Geburtstagsschild (Autodesk Fusion 360 design; units mm, degrees)
Autodesk Fusion 360 part; units mm, degrees
sketch "Sketch2" plane through (0, 0, 0) normal (0, 0, 1) x (1, 0, 0)
  line L0 (0, 0) -> (310, 0)
  line L1 (310, 0) -> (310, 55)
  line L2 (310, 55) -> (0, 55)
  line L3 (0, 55) -> (0, 0)
  dimension "d9" = 310
  dimension "d10" = 55
  constraint horizontal L0
  constraint vertical L1
  constraint horizontal L2
  constraint vertical L3
  constraint coincident L0.start L3.end
  measures "d9" distance of L0.start L0.end
  measures "d10" distance of L0.start L2.end
sketch "Sketch1" plane through (0, 0, 0) normal (0, 0, 1) x (1, 0, 0)
  spline S0 degree 3 poles (59.8411, 26.3898) (55.5097, 27.2397) (53.6137, 32.5028) (55.9347, 36.1804) knots 0 0 0 0 1 1 1 1
  spline S1 degree 3 poles (55.9347, 36.1804) (56.9971, 37.8639) (58.9421, 39.0407) (60.8872, 39.335) knots 0 0 0 0 1 1 1 1
  spline S2 degree 3 poles (60.8872, 39.335) (61.4756, 38.6158) (62.2928, 38.0764) (63.2899, 37.9456) knots 0 0 0 0 1 1 1 1
  spline S3 degree 3 poles (63.2899, 37.9456) (65.2349, 37.7005) (65.856, 39.1225) (64.1071, 39.6782) knots 0 0 0 0 1 1 1 1
  spline S4 degree 3 poles (64.1071, 39.6782) (63.6985, 39.809) (63.1755, 39.907) (62.5707, 39.9561) knots 0 0 0 0 1 1 1 1
  spline S5 degree 3 poles (62.5707, 39.9561) (61.2631, 41.4434) (61.2141, 44.2057) (62.9303, 45.1701) knots 0 0 0 0 1 1 1 1
  spline S6 degree 3 poles (62.9303, 45.1701) (65.856, 46.8373) (66.9021, 43.4212) (65.2022, 43.225) knots 0 0 0 0 1 1 1 1
  spline S7 degree 3 poles (65.2022, 43.225) (64.8753, 43.3721) (64.2542, 43.4048) (64.0254, 43.0943) knots 0 0 0 0 1 1 1 1
  spline S8 degree 3 poles (64.0254, 43.0943) (63.2899, 42.1463) (65.1859, 40.9041) (66.2973, 42.4405) knots 0 0 0 0 1 1 1 1
  spline S9 degree 3 poles (66.2973, 42.4405) (68.2914, 45.1701) (64.7609, 47.442) (61.6881, 45.497) knots 0 0 0 0 1 1 1 1
  spline S10 degree 3 poles (61.6881, 45.497) (59.6286, 44.2057) (59.4815, 41.6723) (60.5112, 39.8907) knots 0 0 0 0 1 1 1 1
  spline S11 degree 3 poles (60.5112, 39.8907) (57.4874, 39.5311) (53.9242, 37.9293) (52.8455, 33.9902) knots 0 0 0 0 1 1 1 1
  spline S12 degree 3 poles (52.8455, 33.9902) (50.3283, 24.7716) (62.8322, 20.7181) (66.232, 29.1357) knots 0 0 0 0 1 1 1 1
  spline S13 degree 3 poles (66.232, 29.1357) (66.706, 30.3126) (66.8367, 32.5355) (65.5291, 33.2547) knots 0 0 0 0 1 1 1 1
  spline S14 degree 3 poles (65.5291, 33.2547) (64.0744, 34.0555) (62.8812, 31.8326) (64.6301, 31.6692) knots 0 0 0 0 1 1 1 1
  spline S15 degree 3 poles (64.6301, 31.6692) (65.4801, 31.3913) (65.856, 30.3616) (65.5291, 29.3809) knots 0 0 0 0 1 1 1 1
  spline S16 degree 3 poles (65.5291, 29.3809) (64.6792, 26.8311) (62.3092, 25.9158) (59.8411, 26.3898) knots 0 0 0 0 1 1 1 1
  spline S17 degree 3 poles (68.7369, 41.9338) (69.3253, 41.7703) (69.9464, 42.2443) (70.1426, 42.9799) knots 0 0 0 0 1 1 1 1
  spline S18 degree 3 poles (70.1426, 42.9799) (70.3224, 43.7154) (69.9955, 44.4509) (69.407, 44.6144) knots 0 0 0 0 1 1 1 1
  spline S19 degree 3 poles (69.407, 44.6144) (68.8186, 44.7778) (68.2139, 44.3201) (68.0014, 43.5846) knots 0 0 0 0 1 1 1 1
  spline S20 degree 3 poles (68.0014, 43.5846) (67.8216, 42.8328) (68.1485, 42.0972) (68.7369, 41.9338) knots 0 0 0 0 1 1 1 1
  spline S21 degree 3 poles (66.0727, 35.0853) (65.6804, 33.794) (66.0727, 32.5028) (67.0861, 32.5028) knots 0 0 0 0 1 1 1 1
  spline S22 degree 3 poles (67.0861, 32.5028) (68.933, 32.5028) (69.8647, 34.8238) (70.3714, 36.7525) knots 0 0 0 0 1 1 1 1
  line L0 (70.3714, 36.7525) -> (69.832, 36.7525)
  spline S23 degree 3 poles (69.832, 36.7525) (69.0311, 34.3171) (68.41, 33.6633) (67.8706, 33.6633) knots 0 0 0 0 1 1 1 1
  spline S24 degree 3 poles (67.8706, 33.6633) (67.4784, 33.6633) (67.5764, 33.9902) (67.7399, 34.5622) knots 0 0 0 0 1 1 1 1
  spline S25 degree 3 poles (67.7399, 34.5622) (67.8543, 34.9382) (69.0965, 39.7599) (69.1782, 40.0378) knots 0 0 0 0 1 1 1 1
  spline S26 degree 3 poles (69.1782, 40.0378) (69.309, 40.5281) (69.1782, 40.806) (68.6715, 40.806) knots 0 0 0 0 1 1 1 1
  line L1 (68.6715, 40.806) -> (67.2495, 40.806)
  spline S27 degree 3 poles (67.2495, 40.806) (67.5764, 40.5118) (67.511, 40.0378) (67.2495, 39.2532) knots 0 0 0 0 1 1 1 1
  spline S28 degree 3 poles (67.2495, 39.2532) (67.1188, 38.8773) (66.1871, 35.4612) (66.0727, 35.0853) knots 0 0 0 0 1 1 1 1
  spline S29 degree 3 poles (73.4638, 32.372) (75.2617, 32.372) (76.2261, 34.8238) (76.8635, 36.7525) knots 0 0 0 0 1 1 1 1
  line L2 (76.8635, 36.7525) -> (76.3732, 36.7525)
  spline S30 degree 3 poles (76.3732, 36.7525) (75.4579, 34.3171) (74.8858, 33.696) (74.4281, 33.696) knots 0 0 0 0 1 1 1 1
  spline S31 degree 3 poles (74.4281, 33.696) (74.0359, 33.696) (73.9868, 33.9902) (74.1176, 34.4315) knots 0 0 0 0 1 1 1 1
  spline S32 degree 3 poles (74.1176, 34.4315) (74.2647, 34.9545) (75.0002, 36.8178) (75.5069, 38.485) knots 0 0 0 0 1 1 1 1
  spline S33 degree 3 poles (75.5069, 38.485) (76.0299, 40.1685) (75.3598, 41.0675) (74.3301, 41.0675) knots 0 0 0 0 1 1 1 1
  spline S34 degree 3 poles (74.3301, 41.0675) (73.5455, 41.0675) (72.7773, 40.5118) (72.1235, 39.4657) knots 0 0 0 0 1 1 1 1
  spline S35 degree 3 poles (72.1235, 39.4657) (72.1725, 40.2993) (71.6332, 40.806) (70.9467, 40.806) knots 0 0 0 0 1 1 1 1
  line L3 (70.9467, 40.806) -> (70.5707, 40.806)
  spline S36 degree 3 poles (70.5707, 40.806) (70.914, 40.4137) (70.7996, 40.0378) (70.5707, 39.2532) knots 0 0 0 0 1 1 1 1
  spline S37 degree 3 poles (70.5707, 39.2532) (70.3909, 38.6158) (69.1487, 34.5296) (68.5767, 32.6335) knots 0 0 0 0 1 1 1 1
  line L4 (68.5767, 32.6335) -> (69.7698, 32.6335)
  spline S38 degree 3 poles (69.7698, 32.6335) (70.2929, 32.6335) (70.5544, 33.0258) (70.6688, 33.5325) knots 0 0 0 0 1 1 1 1
  spline S39 degree 3 poles (70.6688, 33.5325) (70.7505, 33.8758) (71.2245, 35.4449) (71.6332, 36.9649) knots 0 0 0 0 1 1 1 1
  spline S40 degree 3 poles (71.6332, 36.9649) (72.287, 38.91) (73.1205, 40.1685) (73.807, 40.1685) knots 0 0 0 0 1 1 1 1
  spline S41 degree 3 poles (73.807, 40.1685) (74.183, 40.1685) (74.3301, 39.7763) (74.0849, 39.0081) knots 0 0 0 0 1 1 1 1
  spline S42 degree 3 poles (74.0849, 39.0081) (73.807, 38.1091) (72.9081, 36.3765) (72.4177, 34.8238) knots 0 0 0 0 1 1 1 1
  spline S43 degree 3 poles (72.4177, 34.8238) (72.0091, 33.5489) (72.4504, 32.372) (73.4638, 32.372) knots 0 0 0 0 1 1 1 1
  line L5 (77.6468, 26.7494) -> (79.1178, 26.7494)
  spline S44 degree 3 poles (79.1178, 26.7494) (79.6409, 26.7494) (79.9024, 27.1417) (80.0168, 27.6483) knots 0 0 0 0 1 1 1 1
  spline S45 degree 3 poles (80.0168, 27.6483) (80.0822, 27.9099) (80.7523, 30.3616) (81.4715, 32.9604) knots 0 0 0 0 1 1 1 1
  spline S46 degree 3 poles (81.4715, 32.9604) (81.7004, 32.6662) (82.0599, 32.5028) (82.583, 32.5028) knots 0 0 0 0 1 1 1 1
  spline S47 degree 3 poles (82.583, 32.5028) (84.152, 32.5028) (85.7538, 34.4805) (86.3749, 36.7525) knots 0 0 0 0 1 1 1 1
  spline S48 degree 3 poles (86.3749, 36.7525) (87.045, 39.2369) (86.7672, 41.0675) (85.1817, 41.0675) knots 0 0 0 0 1 1 1 1
  spline S49 degree 3 poles (85.1817, 41.0675) (84.3481, 41.0675) (83.6291, 40.4301) (83.0243, 39.4003) knots 0 0 0 0 1 1 1 1
  spline S50 degree 3 poles (83.0243, 39.4003) (83.1224, 40.283) (82.5666, 40.806) (81.8638, 40.806) knots 0 0 0 0 1 1 1 1
  line L6 (81.8638, 40.806) -> (81.4879, 40.806)
  spline S51 degree 3 poles (81.4879, 40.806) (81.8148, 40.4628) (81.7167, 40.0378) (81.4879, 39.2532) knots 0 0 0 0 1 1 1 1
  spline S52 degree 3 poles (81.4879, 39.2532) (81.259, 38.4687) (78.415, 28.4329) (78.2189, 27.7791) knots 0 0 0 0 1 1 1 1
  spline S53 degree 3 poles (78.2189, 27.7791) (78.0391, 27.158) (77.9083, 26.8801) (77.6468, 26.7494) knots 0 0 0 0 1 1 1 1
  line L7 (81.6677, 33.6633) -> (82.4032, 36.3765)
  spline S54 degree 3 poles (82.4032, 36.3765) (82.9753, 38.3706) (83.7435, 39.8907) (84.3972, 40.0378) knots 0 0 0 0 1 1 1 1
  spline S55 degree 3 poles (84.3972, 40.0378) (85.0673, 40.1849) (85.1, 39.1552) (84.5606, 37.1447) knots 0 0 0 0 1 1 1 1
  spline S56 degree 3 poles (84.5606, 37.1447) (84.0703, 35.3468) (83.4329, 33.794) (82.4686, 33.3527) knots 0 0 0 0 1 1 1 1
  spline S57 degree 3 poles (82.4686, 33.3527) (82.0926, 33.1729) (81.7984, 33.32) (81.6677, 33.6633) knots 0 0 0 0 1 1 1 1
  spline S58 degree 3 poles (88.2614, 32.372) (89.0296, 32.372) (89.7161, 33.0422) (90.2554, 33.9738) knots 0 0 0 0 1 1 1 1
  spline S59 degree 3 poles (90.2554, 33.9738) (90.2881, 33.1402) (90.6968, 32.5028) (91.4159, 32.5028) knots 0 0 0 0 1 1 1 1
  spline S60 degree 3 poles (91.4159, 32.5028) (93.0995, 32.5028) (94.0311, 34.8238) (94.5378, 36.7525) knots 0 0 0 0 1 1 1 1
  line L8 (94.5378, 36.7525) -> (93.9984, 36.7525)
  spline S61 degree 3 poles (93.9984, 36.7525) (93.1975, 34.3171) (92.5764, 33.6633) (92.2005, 33.6633) knots 0 0 0 0 1 1 1 1
  spline S62 degree 3 poles (92.2005, 33.6633) (91.8082, 33.6633) (91.8082, 33.9902) (91.9717, 34.5622) knots 0 0 0 0 1 1 1 1
  spline S63 degree 3 poles (91.9717, 34.5622) (92.0697, 34.9055) (93.3283, 39.7109) (93.6061, 40.806) knots 0 0 0 0 1 1 1 1
  line L9 (93.6061, 40.806) -> (92.0534, 40.806)
  spline S64 degree 3 poles (92.0534, 40.806) (92.0043, 40.7079) (91.9226, 40.4301) (91.8082, 40.0378) knots 0 0 0 0 1 1 1 1
  spline S65 degree 3 poles (91.8082, 40.0378) (91.7101, 40.6099) (91.4159, 41.0512) (90.8275, 41.0512) knots 0 0 0 0 1 1 1 1
  spline S66 degree 3 poles (90.8275, 41.0512) (89.8959, 41.0512) (88.1633, 39.6292) (87.3134, 36.7851) knots 0 0 0 0 1 1 1 1
  spline S67 degree 3 poles (87.3134, 36.7851) (86.4634, 33.9411) (87.1336, 32.372) (88.2614, 32.372) knots 0 0 0 0 1 1 1 1
  spline S68 degree 3 poles (88.9479, 36.7525) (89.5036, 38.7302) (90.5333, 39.9397) (91.0563, 39.9397) knots 0 0 0 0 1 1 1 1
  spline S69 degree 3 poles (91.0563, 39.9397) (91.5303, 39.9397) (91.563, 39.335) (91.465, 38.8773) knots 0 0 0 0 1 1 1 1
  spline S70 degree 3 poles (91.465, 38.8773) (91.0727, 37.488) (90.5987, 35.7881) (90.4516, 35.2487) knots 0 0 0 0 1 1 1 1
  spline S71 degree 3 poles (90.4516, 35.2487) (90.2064, 34.6113) (89.8305, 33.9738) (89.3401, 33.9738) knots 0 0 0 0 1 1 1 1
  spline S72 degree 3 poles (89.3401, 33.9738) (88.7517, 33.9738) (88.4412, 34.9382) (88.9479, 36.7525) knots 0 0 0 0 1 1 1 1
  spline S73 degree 3 poles (94.9495, 32.372) (95.7177, 32.372) (96.4042, 33.0422) (96.9436, 33.9738) knots 0 0 0 0 1 1 1 1
  spline S74 degree 3 poles (96.9436, 33.9738) (96.9763, 33.1402) (97.3849, 32.5028) (98.1041, 32.5028) knots 0 0 0 0 1 1 1 1
  spline S75 degree 3 poles (98.1041, 32.5028) (99.7876, 32.5028) (100.7192, 34.8238) (101.2259, 36.7525) knots 0 0 0 0 1 1 1 1
  line L10 (101.2259, 36.7525) -> (100.6866, 36.7525)
  spline S76 degree 3 poles (100.6866, 36.7525) (99.8857, 34.3171) (99.2646, 33.6633) (98.8886, 33.6633) knots 0 0 0 0 1 1 1 1
  spline S77 degree 3 poles (98.8886, 33.6633) (98.4963, 33.6633) (98.4963, 33.9902) (98.6598, 34.5622) knots 0 0 0 0 1 1 1 1
  spline S78 degree 3 poles (98.6598, 34.5622) (98.7579, 34.9055) (100.0164, 39.7109) (100.2943, 40.806) knots 0 0 0 0 1 1 1 1
  line L11 (100.2943, 40.806) -> (98.7415, 40.806)
  spline S79 degree 3 poles (98.7415, 40.806) (98.6925, 40.7079) (98.6108, 40.4301) (98.4963, 40.0378) knots 0 0 0 0 1 1 1 1
  spline S80 degree 3 poles (98.4963, 40.0378) (98.3983, 40.6099) (98.1041, 41.0512) (97.5156, 41.0512) knots 0 0 0 0 1 1 1 1
  spline S81 degree 3 poles (97.5156, 41.0512) (96.584, 41.0512) (94.8514, 39.6292) (94.0015, 36.7851) knots 0 0 0 0 1 1 1 1
  spline S82 degree 3 poles (94.0015, 36.7851) (93.1516, 33.9411) (93.8217, 32.372) (94.9495, 32.372) knots 0 0 0 0 1 1 1 1
  spline S83 degree 3 poles (95.636, 36.7525) (96.1917, 38.7302) (97.2214, 39.9397) (97.7445, 39.9397) knots 0 0 0 0 1 1 1 1
  spline S84 degree 3 poles (97.7445, 39.9397) (98.2185, 39.9397) (98.2512, 39.335) (98.1531, 38.8773) knots 0 0 0 0 1 1 1 1
  spline S85 degree 3 poles (98.1531, 38.8773) (97.7608, 37.488) (97.2868, 35.7881) (97.1397, 35.2487) knots 0 0 0 0 1 1 1 1
  spline S86 degree 3 poles (97.1397, 35.2487) (96.8945, 34.6113) (96.5186, 33.9738) (96.0283, 33.9738) knots 0 0 0 0 1 1 1 1
  spline S87 degree 3 poles (96.0283, 33.9738) (95.4398, 33.9738) (95.1293, 34.9382) (95.636, 36.7525) knots 0 0 0 0 1 1 1 1
  line L12 (99.1692, 32.6335) -> (100.6402, 32.6335)
  spline S88 degree 3 poles (100.6402, 32.6335) (101.1633, 32.6335) (101.4248, 33.0258) (101.5392, 33.5325) knots 0 0 0 0 1 1 1 1
  spline S89 degree 3 poles (101.5392, 33.5325) (101.6209, 33.8758) (102.0949, 35.4612) (102.5199, 36.9976) knots 0 0 0 0 1 1 1 1
  spline S90 degree 3 poles (102.5199, 36.9976) (103.1247, 38.8446) (103.4352, 39.3023) (103.8275, 39.6945) knots 0 0 0 0 1 1 1 1
  spline S91 degree 3 poles (103.8275, 39.6945) (104.089, 39.9561) (104.2361, 39.8743) (104.2525, 39.6455) knots 0 0 0 0 1 1 1 1
  spline S92 degree 3 poles (104.2525, 39.6455) (104.3015, 38.959) (105.3149, 38.8119) (105.6745, 39.5474) knots 0 0 0 0 1 1 1 1
  spline S93 degree 3 poles (105.6745, 39.5474) (106.0504, 40.3156) (105.5601, 41.1165) (104.7918, 41.0839) knots 0 0 0 0 1 1 1 1
  spline S94 degree 3 poles (104.7918, 41.0839) (104.1381, 41.0512) (103.5823, 40.5445) (102.9939, 39.4657) knots 0 0 0 0 1 1 1 1
  spline S95 degree 3 poles (102.9939, 39.4657) (103.0429, 40.2993) (102.5036, 40.806) (101.8171, 40.806) knots 0 0 0 0 1 1 1 1
  line L13 (101.8171, 40.806) -> (101.4411, 40.806)
  spline S96 degree 3 poles (101.4411, 40.806) (101.7354, 40.4791) (101.67, 40.0378) (101.4411, 39.2532) knots 0 0 0 0 1 1 1 1
  spline S97 degree 3 poles (101.4411, 39.2532) (101.2123, 38.4687) (99.9374, 34.3171) (99.7413, 33.6633) knots 0 0 0 0 1 1 1 1
  spline S98 degree 3 poles (99.7413, 33.6633) (99.5615, 33.0422) (99.4307, 32.7643) (99.1692, 32.6335) knots 0 0 0 0 1 1 1 1
  spline S99 degree 3 poles (110.832, 24.9024) (117.8603, 24.1015) (124.0223, 35.0362) (124.8722, 42.3914) knots 0 0 0 0 1 1 1 1
  spline S100 degree 3 poles (124.8722, 42.3914) (125.4607, 39.809) (126.0981, 37.2592) (126.3106, 34.6767) knots 0 0 0 0 1 1 1 1
  spline S101 degree 3 poles (126.3106, 34.6767) (125.6078, 33.32) (125.1011, 31.9307) (124.9703, 30.6885) knots 0 0 0 0 1 1 1 1
  spline S102 degree 3 poles (124.9703, 30.6885) (124.6598, 27.7955) (126.5558, 27.8281) (127.2586, 29.953) knots 0 0 0 0 1 1 1 1
  spline S103 degree 3 poles (127.2586, 29.953) (127.798, 31.6038) (127.9941, 34.0555) (127.9941, 36.2131) knots 0 0 0 0 1 1 1 1
  spline S104 degree 3 poles (127.9941, 36.2131) (129.5959, 38.5994) (131.9986, 41.2473) (134.483, 43.4212) knots 0 0 0 0 1 1 1 1
  spline S105 degree 3 poles (134.483, 43.4212) (133.9764, 42.6203) (133.061, 41.5742) (132.015, 39.2859) knots 0 0 0 0 1 1 1 1
  spline S106 degree 3 poles (132.015, 39.2859) (131.1977, 37.488) (131.0016, 35.7227) (131.2141, 33.7123) knots 0 0 0 0 1 1 1 1
  spline S107 degree 3 poles (131.2141, 33.7123) (131.59, 30.051) (134.8426, 27.5176) (137.229, 29.4463) knots 0 0 0 0 1 1 1 1
  spline S108 degree 3 poles (137.229, 29.4463) (138.226, 30.2635) (136.8857, 31.5548) (136.2646, 30.6068) knots 0 0 0 0 1 1 1 1
  spline S109 degree 3 poles (136.2646, 30.6068) (135.8397, 29.9693) (135.2513, 29.577) (134.6465, 29.7242) knots 0 0 0 0 1 1 1 1
  spline S110 degree 3 poles (134.6465, 29.7242) (133.4043, 30.0347) (132.8159, 31.6202) (133.061, 34.6276) knots 0 0 0 0 1 1 1 1
  spline S111 degree 3 poles (133.061, 34.6276) (133.4697, 39.6292) (136.1339, 45.8239) (140.9883, 47.8016) knots 0 0 0 0 1 1 1 1
  spline S112 degree 3 poles (140.9883, 47.8016) (143.6689, 48.8967) (146.0716, 47.6218) (145.1889, 45.971) knots 0 0 0 0 1 1 1 1
  spline S113 degree 3 poles (145.1889, 45.971) (144.9928, 45.6114) (144.0938, 46.1181) (143.2112, 45.4643) knots 0 0 0 0 1 1 1 1
  spline S114 degree 3 poles (143.2112, 45.4643) (142.1325, 44.6634) (143.2439, 42.8328) (145.4178, 44.2057) knots 0 0 0 0 1 1 1 1
  spline S115 degree 3 poles (145.4178, 44.2057) (146.611, 44.9576) (147.1176, 47.1151) (145.8754, 48.1449) knots 0 0 0 0 1 1 1 1
  spline S116 degree 3 poles (145.8754, 48.1449) (144.6002, 49.1746) (142.8353, 49.0602) (141.3806, 48.5698) knots 0 0 0 0 1 1 1 1
  spline S117 degree 3 poles (141.3806, 48.5698) (136.33, 47.2622) (130.6256, 41.1492) (127.9778, 37.4226) knots 0 0 0 0 1 1 1 1
  line L14 (127.9778, 37.4226) -> (127.9778, 37.4716)
  spline S118 degree 3 poles (127.9778, 37.4716) (127.9124, 39.433) (127.4711, 41.4598) (126.6698, 43.2087) knots 0 0 0 0 1 1 1 1
  spline S119 degree 3 poles (126.6698, 43.2087) (123.6464, 49.8284) (116.945, 49.289) (114.5423, 47.0988) knots 0 0 0 0 1 1 1 1
  spline S120 degree 3 poles (114.5423, 47.0988) (111.1916, 44.0586) (113.3327, 37.8312) (118.5795, 39.3513) knots 0 0 0 0 1 1 1 1
  spline S121 degree 3 poles (118.5795, 39.3513) (121.4071, 40.1685) (119.3477, 43.2414) (117.7786, 41.3454) knots 0 0 0 0 1 1 1 1
  spline S122 degree 3 poles (117.7786, 41.3454) (117.2882, 40.7406) (116.7815, 40.5445) (116.1604, 40.6099) knots 0 0 0 0 1 1 1 1
  spline S123 degree 3 poles (116.1604, 40.6099) (113.3327, 40.8877) (113.0385, 45.0393) (115.1634, 46.6248) knots 0 0 0 0 1 1 1 1
  spline S124 degree 3 poles (115.1634, 46.6248) (118.3506, 49.0111) (122.7964, 47.4584) (124.4309, 43.7317) knots 0 0 0 0 1 1 1 1
  spline S125 degree 3 poles (124.4309, 43.7317) (124.4473, 43.225) (124.3982, 42.702) (124.3165, 42.2117) knots 0 0 0 0 1 1 1 1
  spline S126 degree 3 poles (124.3165, 42.2117) (123.3849, 36.3275) (118.2362, 25.3764) (110.9954, 26.8475) knots 0 0 0 0 1 1 1 1
  spline S127 degree 3 poles (110.9954, 26.8475) (109.7202, 27.109) (109.5567, 25.0495) (110.832, 24.9024) knots 0 0 0 0 1 1 1 1
  spline S128 degree 3 poles (125.7058, 29.2828) (125.428, 30.3943) (125.7058, 31.8) (126.3756, 33.3364) knots 0 0 0 0 1 1 1 1
  line L15 (126.3756, 33.3364) -> (126.3756, 33.1893)
  spline S129 degree 3 poles (126.3756, 33.1893) (126.3923, 31.9307) (126.3433, 30.3453) (125.7058, 29.2828) knots 0 0 0 0 1 1 1 1
  spline S130 degree 3 poles (136.913, 32.372) (137.6812, 32.372) (138.3677, 33.0422) (138.9071, 33.9738) knots 0 0 0 0 1 1 1 1
  spline S131 degree 3 poles (138.9071, 33.9738) (138.9398, 33.1402) (139.3484, 32.5028) (140.0676, 32.5028) knots 0 0 0 0 1 1 1 1
  spline S132 degree 3 poles (140.0676, 32.5028) (141.7511, 32.5028) (142.6827, 34.8238) (143.1894, 36.7525) knots 0 0 0 0 1 1 1 1
  line L16 (143.1894, 36.7525) -> (142.65, 36.7525)
  spline S133 degree 3 poles (142.65, 36.7525) (141.8491, 34.3171) (141.228, 33.6633) (140.8521, 33.6633) knots 0 0 0 0 1 1 1 1
  spline S134 degree 3 poles (140.8521, 33.6633) (140.4598, 33.6633) (140.4598, 33.9902) (140.6233, 34.5622) knots 0 0 0 0 1 1 1 1
  spline S135 degree 3 poles (140.6233, 34.5622) (140.7213, 34.9055) (141.9799, 39.7109) (142.2578, 40.806) knots 0 0 0 0 1 1 1 1
  line L17 (142.2578, 40.806) -> (140.705, 40.806)
  spline S136 degree 3 poles (140.705, 40.806) (140.656, 40.7079) (140.5742, 40.4301) (140.4598, 40.0378) knots 0 0 0 0 1 1 1 1
  spline S137 degree 3 poles (140.4598, 40.0378) (140.3618, 40.6099) (140.0676, 41.0512) (139.4791, 41.0512) knots 0 0 0 0 1 1 1 1
  spline S138 degree 3 poles (139.4791, 41.0512) (138.5475, 41.0512) (136.8149, 39.6292) (135.965, 36.7851) knots 0 0 0 0 1 1 1 1
  spline S139 degree 3 poles (135.965, 36.7851) (135.115, 33.9411) (135.7852, 32.372) (136.913, 32.372) knots 0 0 0 0 1 1 1 1
  spline S140 degree 3 poles (137.5995, 36.7525) (138.1552, 38.7302) (139.1849, 39.9397) (139.708, 39.9397) knots 0 0 0 0 1 1 1 1
  spline S141 degree 3 poles (139.708, 39.9397) (140.182, 39.9397) (140.2147, 39.335) (140.1166, 38.8773) knots 0 0 0 0 1 1 1 1
  spline S142 degree 3 poles (140.1166, 38.8773) (139.7243, 37.488) (139.2503, 35.7881) (139.1032, 35.2487) knots 0 0 0 0 1 1 1 1
  spline S143 degree 3 poles (139.1032, 35.2487) (138.858, 34.6113) (138.4821, 33.9738) (137.9917, 33.9738) knots 0 0 0 0 1 1 1 1
  spline S144 degree 3 poles (137.9917, 33.9738) (137.4033, 33.9738) (137.0928, 34.9382) (137.5995, 36.7525) knots 0 0 0 0 1 1 1 1
  spline S145 degree 3 poles (137.8773, 43.127) (137.8773, 42.5222) (138.384, 41.9828) (138.9888, 41.9828) knots 0 0 0 0 1 1 1 1
  spline S146 degree 3 poles (138.9888, 41.9828) (139.5936, 41.9828) (140.1656, 42.5386) (140.1656, 43.176) knots 0 0 0 0 1 1 1 1
  spline S147 degree 3 poles (140.1656, 43.176) (140.1656, 43.8135) (139.5936, 44.2548) (138.9888, 44.2548) knots 0 0 0 0 1 1 1 1
  spline S148 degree 3 poles (138.9888, 44.2548) (138.384, 44.2548) (137.8773, 43.7481) (137.8773, 43.127) knots 0 0 0 0 1 1 1 1
  spline S149 degree 3 poles (140.754, 43.127) (140.754, 42.5222) (141.2607, 41.9992) (141.8655, 41.9992) knots 0 0 0 0 1 1 1 1
  spline S150 degree 3 poles (141.8655, 41.9992) (142.5356, 41.9992) (142.9933, 42.5549) (142.9933, 43.1433) knots 0 0 0 0 1 1 1 1
  spline S151 degree 3 poles (142.9933, 43.1433) (142.9933, 43.8135) (142.4539, 44.2548) (141.8655, 44.2548) knots 0 0 0 0 1 1 1 1
  spline S152 degree 3 poles (141.8655, 44.2548) (141.2444, 44.2548) (140.754, 43.7481) (140.754, 43.127) knots 0 0 0 0 1 1 1 1
  spline S153 degree 3 poles (143.6011, 32.5028) (144.4184, 32.5028) (145.0722, 33.0422) (145.6115, 33.9411) knots 0 0 0 0 1 1 1 1
  spline S154 degree 3 poles (145.6115, 33.9411) (145.6606, 33.1239) (146.0692, 32.5028) (146.772, 32.5028) knots 0 0 0 0 1 1 1 1
  spline S155 degree 3 poles (146.772, 32.5028) (148.4555, 32.5028) (149.3872, 34.8238) (149.8939, 36.7525) knots 0 0 0 0 1 1 1 1
  line L18 (149.8939, 36.7525) -> (149.3545, 36.7525)
  spline S156 degree 3 poles (149.3545, 36.7525) (148.5536, 34.3171) (147.9325, 33.6633) (147.5566, 33.6633) knots 0 0 0 0 1 1 1 1
  spline S157 degree 3 poles (147.5566, 33.6633) (147.1643, 33.6633) (147.2624, 33.9902) (147.4258, 34.5622) knots 0 0 0 0 1 1 1 1
  spline S158 degree 3 poles (147.4258, 34.5622) (147.5402, 34.9382) (148.7824, 39.7599) (148.8642, 40.0378) knots 0 0 0 0 1 1 1 1
  spline S159 degree 3 poles (148.8642, 40.0378) (148.9949, 40.5281) (148.8642, 40.806) (148.3575, 40.806) knots 0 0 0 0 1 1 1 1
  line L19 (148.3575, 40.806) -> (146.9355, 40.806)
  spline S160 degree 3 poles (146.9355, 40.806) (147.2624, 40.4464) (147.197, 40.0378) (146.9355, 39.2532) knots 0 0 0 0 1 1 1 1
  spline S161 degree 3 poles (146.9355, 39.2532) (146.8701, 39.0571) (146.5922, 38.0437) (146.3144, 37.063) knots 0 0 0 0 1 1 1 1
  spline S162 degree 3 poles (146.3144, 37.063) (145.4317, 34.219) (144.925, 33.6633) (144.3203, 33.6633) knots 0 0 0 0 1 1 1 1
  spline S163 degree 3 poles (144.3203, 33.6633) (143.928, 33.6633) (143.6665, 33.9902) (143.8299, 34.5622) knots 0 0 0 0 1 1 1 1
  spline S164 degree 3 poles (143.8299, 34.5622) (143.9444, 34.9382) (145.1866, 39.7599) (145.2683, 40.0378) knots 0 0 0 0 1 1 1 1
  spline S165 degree 3 poles (145.2683, 40.0378) (145.399, 40.5281) (145.2683, 40.806) (144.7616, 40.806) knots 0 0 0 0 1 1 1 1
  line L20 (144.7616, 40.806) -> (143.3396, 40.806)
  spline S166 degree 3 poles (143.3396, 40.806) (143.6665, 40.4464) (143.6011, 40.0378) (143.3396, 39.2532) knots 0 0 0 0 1 1 1 1
  spline S167 degree 3 poles (143.3396, 39.2532) (143.2088, 38.8773) (142.2772, 35.4612) (142.1628, 35.0853) knots 0 0 0 0 1 1 1 1
  spline S168 degree 3 poles (142.1628, 35.0853) (141.7705, 33.794) (142.1628, 32.5028) (143.6011, 32.5028) knots 0 0 0 0 1 1 1 1
  spline S169 degree 3 poles (150.9424, 32.3884) (152.6422, 32.3884) (153.8027, 33.8594) (153.7046, 35.2487) knots 0 0 0 0 1 1 1 1
  spline S170 degree 3 poles (153.7046, 35.2487) (153.5739, 37.063) (152.0702, 38.0764) (151.825, 39.1878) knots 0 0 0 0 1 1 1 1
  spline S171 degree 3 poles (151.825, 39.1878) (151.6125, 40.1522) (152.1028, 40.757) (152.6749, 40.7079) knots 0 0 0 0 1 1 1 1
  spline S172 degree 3 poles (152.6749, 40.7079) (153.2143, 40.6589) (153.2306, 39.9887) (153.1162, 39.4003) knots 0 0 0 0 1 1 1 1
  spline S173 degree 3 poles (153.1162, 39.4003) (152.8874, 38.1908) (154.8324, 38.2235) (154.5873, 39.6945) knots 0 0 0 0 1 1 1 1
  spline S174 degree 3 poles (154.5873, 39.6945) (154.4238, 40.6589) (153.6556, 41.1656) (152.5442, 41.1819) knots 0 0 0 0 1 1 1 1
  spline S175 degree 3 poles (152.5442, 41.1819) (151.4327, 41.1983) (150.1088, 40.283) (150.3703, 38.5014) knots 0 0 0 0 1 1 1 1
  spline S176 degree 3 poles (150.3703, 38.5014) (150.5991, 36.9323) (152.3971, 35.7718) (152.1846, 34.2353) knots 0 0 0 0 1 1 1 1
  spline S177 degree 3 poles (152.1846, 34.2353) (152.0538, 33.3527) (151.5798, 33.0095) (150.9587, 33.0095) knots 0 0 0 0 1 1 1 1
  spline S178 degree 3 poles (150.9587, 33.0095) (149.8473, 33.0095) (149.3242, 34.1209) (150.1741, 35.5429) knots 0 0 0 0 1 1 1 1
  spline S179 degree 3 poles (150.1741, 35.5429) (150.926, 36.7851) (149.2098, 37.3736) (148.7521, 36.1314) knots 0 0 0 0 1 1 1 1
  spline S180 degree 3 poles (148.7521, 36.1314) (148.2291, 34.7093) (148.7031, 32.3884) (150.9424, 32.3884) knots 0 0 0 0 1 1 1 1
  spline S181 degree 3 poles (156.7942, 32.5028) (158.5758, 32.5028) (160.1939, 34.3824) (160.815, 36.7525) knots 0 0 0 0 1 1 1 1
  line L21 (160.815, 36.7525) -> (160.2756, 36.7525)
  spline S182 degree 3 poles (160.2756, 36.7525) (159.4911, 34.3498) (158.2325, 33.5325) (157.3499, 33.696) knots 0 0 0 0 1 1 1 1
  spline S183 degree 3 poles (157.3499, 33.696) (156.549, 33.8431) (156.1567, 35.0362) (156.3855, 36.3765) knots 0 0 0 0 1 1 1 1
  spline S184 degree 3 poles (156.3855, 36.3765) (160.1612, 36.0169) (161.24, 41.0675) (158.5758, 41.0675) knots 0 0 0 0 1 1 1 1
  spline S185 degree 3 poles (158.5758, 41.0675) (156.6798, 41.0675) (155.1597, 38.6812) (154.7674, 36.7198) knots 0 0 0 0 1 1 1 1
  spline S186 degree 3 poles (154.7674, 36.7198) (154.2934, 34.3824) (154.9635, 32.5028) (156.7942, 32.5028) knots 0 0 0 0 1 1 1 1
  spline S187 degree 3 poles (156.4836, 36.8669) (156.974, 38.91) (158.02, 40.5445) (158.8373, 40.5445) knots 0 0 0 0 1 1 1 1
  spline S188 degree 3 poles (158.8373, 40.5445) (159.6055, 40.5445) (158.919, 37.2428) (156.4836, 36.8669) knots 0 0 0 0 1 1 1 1
  spline S189 degree 3 poles (76.4934, 3.3435) (77.7847, 3.3435) (79.2067, 4.6511) (79.7624, 6.7596) knots 0 0 0 0 1 1 1 1
  spline S190 degree 3 poles (79.7624, 6.7596) (80.1547, 7.9201) (81.2661, 12.9053) (81.8872, 15.6348) knots 0 0 0 0 1 1 1 1
  line L22 (81.8872, 15.6348) -> (82.9987, 15.6348)
  line L23 (82.9987, 15.6348) -> (83.1621, 16.2886)
  line L24 (83.1621, 16.2886) -> (82.0507, 16.2886)
  line L25 (82.0507, 16.2886) -> (82.2795, 17.2693)
  spline S191 degree 3 poles (82.2795, 17.2693) (82.6554, 18.7404) (83.2112, 19.5576) (83.8813, 19.8355) knots 0 0 0 0 1 1 1 1
  spline S192 degree 3 poles (83.8813, 19.8355) (84.2409, 19.9826) (84.4207, 19.7701) (84.1591, 19.4269) knots 0 0 0 0 1 1 1 1
  spline S193 degree 3 poles (84.1591, 19.4269) (83.6525, 18.7731) (84.7149, 18.0049) (85.1562, 18.8548) knots 0 0 0 0 1 1 1 1
  spline S194 degree 3 poles (85.1562, 18.8548) (85.4994, 19.5249) (85.0091, 20.4076) (83.8323, 20.4076) knots 0 0 0 0 1 1 1 1
  spline S195 degree 3 poles (83.8323, 20.4076) (82.541, 20.4076) (81.2334, 19.3288) (80.6777, 17.2203) knots 0 0 0 0 1 1 1 1
  spline S196 degree 3 poles (80.6777, 17.2203) (80.6287, 17.0405) (80.5633, 16.7463) (80.4489, 16.2886) knots 0 0 0 0 1 1 1 1
  line L26 (80.4489, 16.2886) -> (79.648, 16.2886)
  line L27 (79.648, 16.2886) -> (79.4845, 15.6348)
  line L28 (79.4845, 15.6348) -> (80.2854, 15.6348)
  spline S197 degree 3 poles (80.2854, 15.6348) (79.9095, 14.1148) (79.2394, 11.3852) (77.9808, 6.4817) knots 0 0 0 0 1 1 1 1
  spline S198 degree 3 poles (77.9808, 6.4817) (77.6049, 5.0107) (77.1145, 4.1934) (76.4444, 3.9156) knots 0 0 0 0 1 1 1 1
  spline S199 degree 3 poles (76.4444, 3.9156) (76.0848, 3.7684) (75.905, 3.9809) (76.1665, 4.3242) knots 0 0 0 0 1 1 1 1
  spline S200 degree 3 poles (76.1665, 4.3242) (76.6732, 4.978) (75.6108, 5.7462) (75.1695, 4.8963) knots 0 0 0 0 1 1 1 1
  spline S201 degree 3 poles (75.1695, 4.8963) (74.8262, 4.2261) (75.3166, 3.3435) (76.4934, 3.3435) knots 0 0 0 0 1 1 1 1
  spline S202 degree 3 poles (83.401, 7.9854) (84.2184, 7.9854) (84.8722, 8.5248) (85.4116, 9.4238) knots 0 0 0 0 1 1 1 1
  spline S203 degree 3 poles (85.4116, 9.4238) (85.4606, 8.6065) (85.8692, 7.9854) (86.5721, 7.9854) knots 0 0 0 0 1 1 1 1
  spline S204 degree 3 poles (86.5721, 7.9854) (88.2556, 7.9854) (89.1872, 10.3064) (89.6939, 12.2351) knots 0 0 0 0 1 1 1 1
  line L29 (89.6939, 12.2351) -> (89.1545, 12.2351)
  spline S205 degree 3 poles (89.1545, 12.2351) (88.3536, 9.7997) (87.7325, 9.1459) (87.3566, 9.1459) knots 0 0 0 0 1 1 1 1
  spline S206 degree 3 poles (87.3566, 9.1459) (86.9643, 9.1459) (87.0624, 9.4728) (87.2258, 10.0449) knots 0 0 0 0 1 1 1 1
  spline S207 degree 3 poles (87.2258, 10.0449) (87.3403, 10.4208) (88.5825, 15.2426) (88.6642, 15.5204) knots 0 0 0 0 1 1 1 1
  spline S208 degree 3 poles (88.6642, 15.5204) (88.795, 16.0108) (88.6642, 16.2886) (88.1575, 16.2886) knots 0 0 0 0 1 1 1 1
  line L30 (88.1575, 16.2886) -> (86.7355, 16.2886)
  spline S209 degree 3 poles (86.7355, 16.2886) (87.0624, 15.9291) (86.997, 15.5204) (86.7355, 14.7359) knots 0 0 0 0 1 1 1 1
  spline S210 degree 3 poles (86.7355, 14.7359) (86.6701, 14.5397) (86.3923, 13.5264) (86.1144, 12.5457) knots 0 0 0 0 1 1 1 1
  spline S211 degree 3 poles (86.1144, 12.5457) (85.2318, 9.7016) (84.7251, 9.1459) (84.1203, 9.1459) knots 0 0 0 0 1 1 1 1
  spline S212 degree 3 poles (84.1203, 9.1459) (83.7279, 9.1459) (83.4664, 9.4728) (83.6299, 10.0449) knots 0 0 0 0 1 1 1 1
  spline S213 degree 3 poles (83.6299, 10.0449) (83.7443, 10.4208) (84.9866, 15.2426) (85.0683, 15.5204) knots 0 0 0 0 1 1 1 1
  spline S214 degree 3 poles (85.0683, 15.5204) (85.1991, 16.0108) (85.0683, 16.2886) (84.5616, 16.2886) knots 0 0 0 0 1 1 1 1
  line L31 (84.5616, 16.2886) -> (83.1395, 16.2886)
  spline S215 degree 3 poles (83.1395, 16.2886) (83.4664, 15.9291) (83.401, 15.5204) (83.1395, 14.7359) knots 0 0 0 0 1 1 1 1
  spline S216 degree 3 poles (83.1395, 14.7359) (83.0088, 14.3599) (82.0771, 10.9439) (81.9627, 10.5679) knots 0 0 0 0 1 1 1 1
  spline S217 degree 3 poles (81.9627, 10.5679) (81.5704, 9.2767) (81.9627, 7.9854) (83.401, 7.9854) knots 0 0 0 0 1 1 1 1
  spline S218 degree 3 poles (83.5972, 18.201) (83.5972, 17.5962) (84.104, 17.0569) (84.7087, 17.0569) knots 0 0 0 0 1 1 1 1
  spline S219 degree 3 poles (84.7087, 17.0569) (85.3135, 17.0569) (85.8856, 17.6126) (85.8856, 18.25) knots 0 0 0 0 1 1 1 1
  spline S220 degree 3 poles (85.8856, 18.25) (85.8856, 18.8875) (85.3135, 19.3288) (84.7087, 19.3288) knots 0 0 0 0 1 1 1 1
  spline S221 degree 3 poles (84.7087, 19.3288) (84.104, 19.3288) (83.5972, 18.8221) (83.5972, 18.201) knots 0 0 0 0 1 1 1 1
  spline S222 degree 3 poles (86.474, 18.201) (86.474, 17.5962) (86.9807, 17.0732) (87.5854, 17.0732) knots 0 0 0 0 1 1 1 1
  spline S223 degree 3 poles (87.5854, 17.0732) (88.2556, 17.0732) (88.7132, 17.6289) (88.7132, 18.2173) knots 0 0 0 0 1 1 1 1
  spline S224 degree 3 poles (88.7132, 18.2173) (88.7132, 18.8875) (88.1739, 19.3288) (87.5854, 19.3288) knots 0 0 0 0 1 1 1 1
  spline S225 degree 3 poles (87.5854, 19.3288) (86.9643, 19.3288) (86.474, 18.8221) (86.474, 18.201) knots 0 0 0 0 1 1 1 1
  line L32 (87.6369, 8.1162) -> (89.1079, 8.1162)
  spline S226 degree 3 poles (89.1079, 8.1162) (89.6309, 8.1162) (89.8925, 8.5085) (90.0069, 9.0152) knots 0 0 0 0 1 1 1 1
  spline S227 degree 3 poles (90.0069, 9.0152) (90.0886, 9.3584) (90.5626, 10.9439) (90.9876, 12.4803) knots 0 0 0 0 1 1 1 1
  spline S228 degree 3 poles (90.9876, 12.4803) (91.5923, 14.3273) (91.9029, 14.7849) (92.2952, 15.1772) knots 0 0 0 0 1 1 1 1
  spline S229 degree 3 poles (92.2952, 15.1772) (92.5567, 15.4387) (92.7038, 15.357) (92.7201, 15.1282) knots 0 0 0 0 1 1 1 1
  spline S230 degree 3 poles (92.7201, 15.1282) (92.7692, 14.4417) (93.7825, 14.2946) (94.1421, 15.0301) knots 0 0 0 0 1 1 1 1
  spline S231 degree 3 poles (94.1421, 15.0301) (94.5181, 15.7983) (94.0277, 16.5992) (93.2595, 16.5665) knots 0 0 0 0 1 1 1 1
  spline S232 degree 3 poles (93.2595, 16.5665) (92.6057, 16.5338) (92.05, 16.0271) (91.4616, 14.9484) knots 0 0 0 0 1 1 1 1
  spline S233 degree 3 poles (91.4616, 14.9484) (91.5106, 15.782) (90.9712, 16.2886) (90.2847, 16.2886) knots 0 0 0 0 1 1 1 1
  line L33 (90.2847, 16.2886) -> (89.9088, 16.2886)
  spline S234 degree 3 poles (89.9088, 16.2886) (90.203, 15.9617) (90.1376, 15.5204) (89.9088, 14.7359) knots 0 0 0 0 1 1 1 1
  spline S235 degree 3 poles (89.9088, 14.7359) (89.68, 13.9513) (88.4051, 9.7997) (88.2089, 9.1459) knots 0 0 0 0 1 1 1 1
  spline S236 degree 3 poles (88.2089, 9.1459) (88.0291, 8.5248) (87.8984, 8.247) (87.6369, 8.1162) knots 0 0 0 0 1 1 1 1
  spline S237 degree 3 poles (105.4286, 3.6377) (112.3916, 6.1058) (113.3886, 14.3599) (115.4317, 20.522) knots 0 0 0 0 1 1 1 1
  spline S238 degree 3 poles (115.4317, 20.522) (115.8403, 21.7805) (116.3797, 23.1535) (117.6056, 23.7092) knots 0 0 0 0 1 1 1 1
  line L34 (117.6056, 23.7092) -> (117.6219, 23.7092)
  line L35 (117.6219, 23.7092) -> (117.6546, 23.7256)
  spline S239 degree 3 poles (117.6546, 23.7256) (118.145, 23.8727) (117.8181, 24.6082) (117.3767, 24.4121) knots 0 0 0 0 1 1 1 1
  spline S240 degree 3 poles (117.3767, 24.4121) (116.5595, 24.0525) (115.7259, 23.8563) (114.8596, 23.6602) knots 0 0 0 0 1 1 1 1
  spline S241 degree 3 poles (114.8596, 23.6602) (111.9829, 23.0064) (109.1716, 23.366) (106.393, 22.2218) knots 0 0 0 0 1 1 1 1
  spline S242 degree 3 poles (106.393, 22.2218) (103.8595, 21.1758) (102.3394, 17.776) (104.2518, 15.3243) knots 0 0 0 0 1 1 1 1
  spline S243 degree 3 poles (104.2518, 15.3243) (105.1671, 14.1475) (107.9294, 14.507) (107.5371, 16.1088) knots 0 0 0 0 1 1 1 1
  spline S244 degree 3 poles (107.5371, 16.1088) (107.39, 16.7626) (106.6055, 16.6809) (106.1968, 16.2396) knots 0 0 0 0 1 1 1 1
  spline S245 degree 3 poles (106.1968, 16.2396) (104.3989, 14.3109) (103.549, 17.5635) (104.6931, 19.1163) knots 0 0 0 0 1 1 1 1
  spline S246 degree 3 poles (104.6931, 19.1163) (106.1478, 21.0777) (107.9621, 21.3719) (109.8744, 21.8786) knots 0 0 0 0 1 1 1 1
  spline S247 degree 3 poles (109.8744, 21.8786) (111.8522, 22.4016) (113.9607, 22.7939) (115.9711, 23.2843) knots 0 0 0 0 1 1 1 1
  spline S248 degree 3 poles (115.9711, 23.2843) (111.6233, 18.7404) (111.6887, 12.0226) (108.6649, 7.0211) knots 0 0 0 0 1 1 1 1
  spline S249 degree 3 poles (108.6649, 7.0211) (107.0958, 4.4222) (103.7124, 3.082) (101.0318, 4.7165) knots 0 0 0 0 1 1 1 1
  spline S250 degree 3 poles (101.0318, 4.7165) (99.0051, 5.9423) (99.1685, 8.6556) (101.2607, 8.819) knots 0 0 0 0 1 1 1 1
  spline S251 degree 3 poles (101.2607, 8.819) (102.7644, 8.9498) (102.2577, 10.8621) (100.7213, 10.666) knots 0 0 0 0 1 1 1 1
  spline S252 degree 3 poles (100.7213, 10.666) (99.7569, 10.5516) (98.8743, 9.669) (98.5965, 8.7046) knots 0 0 0 0 1 1 1 1
  spline S253 degree 3 poles (98.5965, 8.7046) (97.436, 4.6674) (102.0943, 2.4609) (105.4286, 3.6377) knots 0 0 0 0 1 1 1 1
  spline S254 degree 3 poles (118.5001, 7.8547) (120.2981, 7.8547) (121.2624, 10.3064) (121.8999, 12.2351) knots 0 0 0 0 1 1 1 1
  line L36 (121.8999, 12.2351) -> (121.4095, 12.2351)
  spline S255 degree 3 poles (121.4095, 12.2351) (120.4942, 9.7997) (119.9221, 9.1786) (119.4645, 9.1786) knots 0 0 0 0 1 1 1 1
  spline S256 degree 3 poles (119.4645, 9.1786) (119.0722, 9.1786) (119.0231, 9.4728) (119.1539, 9.9141) knots 0 0 0 0 1 1 1 1
  spline S257 degree 3 poles (119.1539, 9.9141) (119.301, 10.4372) (120.0365, 12.3005) (120.5432, 13.9677) knots 0 0 0 0 1 1 1 1
  spline S258 degree 3 poles (120.5432, 13.9677) (121.0663, 15.6512) (120.3961, 16.5502) (119.3664, 16.5502) knots 0 0 0 0 1 1 1 1
  spline S259 degree 3 poles (119.3664, 16.5502) (118.5818, 16.5502) (117.8136, 15.9944) (117.1598, 14.9484) knots 0 0 0 0 1 1 1 1
  spline S260 degree 3 poles (117.1598, 14.9484) (117.2089, 15.782) (116.6695, 16.2886) (115.983, 16.2886) knots 0 0 0 0 1 1 1 1
  line L37 (115.983, 16.2886) -> (115.6071, 16.2886)
  spline S261 degree 3 poles (115.6071, 16.2886) (115.9503, 15.8964) (115.8359, 15.5204) (115.6071, 14.7359) knots 0 0 0 0 1 1 1 1
  spline S262 degree 3 poles (115.6071, 14.7359) (115.4273, 14.0984) (114.1851, 10.0122) (113.613, 8.1162) knots 0 0 0 0 1 1 1 1
  line L38 (113.613, 8.1162) -> (114.8062, 8.1162)
  spline S263 degree 3 poles (114.8062, 8.1162) (115.3292, 8.1162) (115.5907, 8.5085) (115.7051, 9.0152) knots 0 0 0 0 1 1 1 1
  spline S264 degree 3 poles (115.7051, 9.0152) (115.7869, 9.3584) (116.2609, 10.9275) (116.6695, 12.4476) knots 0 0 0 0 1 1 1 1
  spline S265 degree 3 poles (116.6695, 12.4476) (117.3233, 14.3926) (118.1569, 15.6512) (118.8434, 15.6512) knots 0 0 0 0 1 1 1 1
  spline S266 degree 3 poles (118.8434, 15.6512) (119.2193, 15.6512) (119.3664, 15.2589) (119.1212, 14.4907) knots 0 0 0 0 1 1 1 1
  spline S267 degree 3 poles (119.1212, 14.4907) (118.8434, 13.5917) (117.9444, 11.8592) (117.454, 10.3064) knots 0 0 0 0 1 1 1 1
  spline S268 degree 3 poles (117.454, 10.3064) (117.0454, 9.0315) (117.4867, 7.8547) (118.5001, 7.8547) knots 0 0 0 0 1 1 1 1
  spline S269 degree 3 poles (133.168, 3.131) (137.434, 2.7224) (138.3166, 5.3703) (137.6628, 6.4163) knots 0 0 0 0 1 1 1 1
  spline S270 degree 3 poles (137.6628, 6.4163) (136.7965, 7.7893) (135.0967, 6.0077) (136.96, 5.0924) knots 0 0 0 0 1 1 1 1
  spline S271 degree 3 poles (136.96, 5.0924) (136.96, 4.3242) (135.3745, 3.9646) (130.7326, 5.2558) knots 0 0 0 0 1 1 1 1
  spline S272 degree 3 poles (130.7326, 5.2558) (128.9346, 5.7625) (127.1367, 6.6125) (125.3224, 7.0701) knots 0 0 0 0 1 1 1 1
  line L39 (125.3224, 7.0701) -> (127.8068, 16.2886)
  line L40 (127.8068, 16.2886) -> (126.107, 16.2886)
  line L41 (126.107, 16.2886) -> (125.8945, 15.5368)
  spline S273 degree 3 poles (125.8945, 15.5368) (125.8128, 16.0925) (125.5185, 16.5338) (124.9301, 16.5338) knots 0 0 0 0 1 1 1 1
  spline S274 degree 3 poles (124.9301, 16.5338) (123.9985, 16.5338) (122.2659, 15.1118) (121.416, 12.2678) knots 0 0 0 0 1 1 1 1
  spline S275 degree 3 poles (121.416, 12.2678) (120.566, 9.4238) (121.2362, 7.8547) (122.364, 7.8547) knots 0 0 0 0 1 1 1 1
  spline S276 degree 3 poles (122.364, 7.8547) (123.0341, 7.8547) (123.6552, 8.3777) (124.1619, 9.1459) knots 0 0 0 0 1 1 1 1
  line L42 (124.1619, 9.1459) -> (123.6225, 7.1682)
  spline S277 degree 3 poles (123.6225, 7.1682) (122.838, 7.1355) (122.0534, 6.9394) (121.2525, 6.5471) knots 0 0 0 0 1 1 1 1
  spline S278 degree 3 poles (121.2525, 6.5471) (120.2391, 6.0404) (119.7651, 5.076) (119.6998, 4.3569) knots 0 0 0 0 1 1 1 1
  spline S279 degree 3 poles (119.6998, 4.3569) (119.4709, 1.6926) (123.7533, 1.4475) (124.9138, 5.5337) knots 0 0 0 0 1 1 1 1
  line L43 (124.9138, 5.5337) -> (125.0936, 6.1711)
  spline S280 degree 3 poles (125.0936, 6.1711) (126.7444, 5.5337) (129.6701, 3.4579) (133.168, 3.131) knots 0 0 0 0 1 1 1 1
  spline S281 degree 3 poles (121.1871, 4.3405) (121.5304, 5.7789) (122.2823, 6.5144) (123.5081, 6.4654) knots 0 0 0 0 1 1 1 1
  line L44 (123.5081, 6.4654) -> (123.2629, 5.55)
  spline S282 degree 3 poles (123.2629, 5.55) (122.364, 2.2157) (120.7622, 2.5426) (121.1871, 4.3405) knots 0 0 0 0 1 1 1 1
  spline S283 degree 3 poles (123.0505, 12.2351) (123.6062, 14.2128) (124.6359, 15.4224) (125.159, 15.4224) knots 0 0 0 0 1 1 1 1
  spline S284 degree 3 poles (125.159, 15.4224) (125.682, 15.4224) (125.6657, 14.6868) (125.5349, 14.2128) knots 0 0 0 0 1 1 1 1
  line L45 (125.5349, 14.2128) -> (125.5349, 14.1965)
  line L46 (125.5349, 14.1965) -> (124.7503, 11.2708)
  line L47 (124.7503, 11.2708) -> (124.685, 11.1073)
  spline S285 degree 3 poles (124.685, 11.1073) (124.4398, 10.3881) (124.0312, 9.4565) (123.4427, 9.4565) knots 0 0 0 0 1 1 1 1
  spline S286 degree 3 poles (123.4427, 9.4565) (122.8543, 9.4565) (122.5438, 10.4208) (123.0505, 12.2351) knots 0 0 0 0 1 1 1 1
  spline S287 degree 3 poles (129.7628, 7.9854) (131.5444, 7.9854) (133.1625, 9.8651) (133.7836, 12.2351) knots 0 0 0 0 1 1 1 1
  line L48 (133.7836, 12.2351) -> (133.2442, 12.2351)
  spline S288 degree 3 poles (133.2442, 12.2351) (132.4597, 9.8324) (131.2011, 9.0152) (130.3185, 9.1786) knots 0 0 0 0 1 1 1 1
  spline S289 degree 3 poles (130.3185, 9.1786) (129.5176, 9.3257) (129.1253, 10.5189) (129.3541, 11.8592) knots 0 0 0 0 1 1 1 1
  spline S290 degree 3 poles (129.3541, 11.8592) (133.1298, 11.4996) (134.2086, 16.5502) (131.5444, 16.5502) knots 0 0 0 0 1 1 1 1
  spline S291 degree 3 poles (131.5444, 16.5502) (129.6484, 16.5502) (128.1283, 14.1638) (127.736, 12.2024) knots 0 0 0 0 1 1 1 1
  spline S292 degree 3 poles (127.736, 12.2024) (127.262, 9.8651) (127.9321, 7.9854) (129.7628, 7.9854) knots 0 0 0 0 1 1 1 1
  spline S293 degree 3 poles (129.4522, 12.3495) (129.9426, 14.3926) (130.9886, 16.0271) (131.8059, 16.0271) knots 0 0 0 0 1 1 1 1
  spline S294 degree 3 poles (131.8059, 16.0271) (132.5741, 16.0271) (131.8876, 12.7255) (129.4522, 12.3495) knots 0 0 0 0 1 1 1 1
sketch "Sketch3" plane through (0, 0, 0) normal (0, 0, 1) x (1, 0, 0)
  line L0 (46.9601, 53.7573) -> (166.5514, 53.7573)
  line L1 (166.5514, 53.7573) -> (166.5514, -1.6336)
  line L2 (166.5514, -1.6336) -> (46.9601, -1.6336)
  line L3 (46.9601, -1.6336) -> (46.9601, 53.7573)
  constraint horizontal L0
  constraint vertical L1
  constraint horizontal L2
  constraint vertical L3
sketch "Sketch4" plane through (0, 0, 0) normal (0, 0, 1) x (1, 0, 0)
  spline S0 degree 3 poles (61.44, 19.1895) (57.6876, 19.1895) (54.6352, 16.137) (54.6352, 12.3846) knots 0 0 0 0 1 1 1 1
  spline S1 degree 3 poles (54.6352, 12.3846) (54.6352, 8.6323) (57.6876, 5.5798) (61.44, 5.5798) knots 0 0 0 0 1 1 1 1
  spline S2 degree 3 poles (61.44, 5.5798) (65.1924, 5.5798) (68.2449, 8.6323) (68.2449, 12.3846) knots 0 0 0 0 1 1 1 1
  spline S3 degree 3 poles (68.2449, 12.3846) (68.2449, 16.137) (65.1924, 19.1895) (61.44, 19.1895) knots 0 0 0 0 1 1 1 1
  spline S4 degree 3 poles (61.44, 6.713) (58.3126, 6.713) (55.7684, 9.2572) (55.7684, 12.3846) knots 0 0 0 0 1 1 1 1
  spline S5 degree 3 poles (55.7684, 12.3846) (55.7684, 15.5121) (58.3126, 18.0563) (61.44, 18.0563) knots 0 0 0 0 1 1 1 1
  spline S6 degree 3 poles (61.44, 18.0563) (64.5675, 18.0563) (67.1117, 15.5121) (67.1117, 12.3846) knots 0 0 0 0 1 1 1 1
  spline S7 degree 3 poles (67.1117, 12.3846) (67.1117, 9.2572) (64.5675, 6.713) (61.44, 6.713) knots 0 0 0 0 1 1 1 1
  line L0 (61.7956, 13.2512) -> (61.7956, 15.0983)
  spline S8 degree 3 poles (61.7956, 15.0983) (62.1011, 14.9649) (62.2899, 14.715) (62.3622, 14.3428) knots 0 0 0 0 1 1 1 1
  line L1 (62.3622, 14.3428) -> (63.5565, 14.4983)
  spline S9 degree 3 poles (63.5565, 14.4983) (63.4759, 14.9705) (63.2843, 15.3482) (62.9899, 15.6288) knots 0 0 0 0 1 1 1 1
  spline S10 degree 3 poles (62.9899, 15.6288) (62.6927, 15.9121) (62.2955, 16.0815) (61.7956, 16.1426) knots 0 0 0 0 1 1 1 1
  line L2 (61.7956, 16.1426) -> (61.7956, 16.6092)
  line L3 (61.7956, 16.6092) -> (61.1095, 16.6092)
  line L4 (61.1095, 16.6092) -> (61.1095, 16.1426)
  spline S11 degree 3 poles (61.1095, 16.1426) (60.5679, 16.0898) (60.1346, 15.8871) (59.8069, 15.5343) knots 0 0 0 0 1 1 1 1
  spline S12 degree 3 poles (59.8069, 15.5343) (59.4819, 15.1844) (59.318, 14.7483) (59.318, 14.2317) knots 0 0 0 0 1 1 1 1
  spline S13 degree 3 poles (59.318, 14.2317) (59.318, 13.7206) (59.4625, 13.2873) (59.7513, 12.929) knots 0 0 0 0 1 1 1 1
  spline S14 degree 3 poles (59.7513, 12.929) (60.0402, 12.5707) (60.4929, 12.3041) (61.1095, 12.1291) knots 0 0 0 0 1 1 1 1
  line L5 (61.1095, 12.1291) -> (61.1095, 10.1488)
  spline S15 degree 3 poles (61.1095, 10.1488) (60.9401, 10.2293) (60.7845, 10.3626) (60.6457, 10.5459) knots 0 0 0 0 1 1 1 1
  spline S16 degree 3 poles (60.6457, 10.5459) (60.5068, 10.7293) (60.4124, 10.9459) (60.3624, 11.1987) knots 0 0 0 0 1 1 1 1
  line L6 (60.3624, 11.1987) -> (59.1292, 11.0653)
  spline S17 degree 3 poles (59.1292, 11.0653) (59.2236, 10.446) (59.4402, 9.9655) (59.7819, 9.6238) knots 0 0 0 0 1 1 1 1
  spline S18 degree 3 poles (59.7819, 9.6238) (60.1235, 9.2822) (60.5651, 9.0794) (61.1095, 9.0156) knots 0 0 0 0 1 1 1 1
  line L7 (61.1095, 9.0156) -> (61.1095, 8.1545)
  line L8 (61.1095, 8.1545) -> (61.7956, 8.1545)
  line L9 (61.7956, 8.1545) -> (61.7956, 9.0378)
  spline S19 degree 3 poles (61.7956, 9.0378) (62.4094, 9.1267) (62.8899, 9.3655) (63.2343, 9.7571) knots 0 0 0 0 1 1 1 1
  spline S20 degree 3 poles (63.2343, 9.7571) (63.5787, 10.1488) (63.7509, 10.6293) (63.7509, 11.1987) knots 0 0 0 0 1 1 1 1
  spline S21 degree 3 poles (63.7509, 11.1987) (63.7509, 11.7097) (63.6148, 12.1263) (63.3398, 12.4541) knots 0 0 0 0 1 1 1 1
  spline S22 degree 3 poles (63.3398, 12.4541) (63.0649, 12.7818) (62.551, 13.0457) (61.7956, 13.2512) knots 0 0 0 0 1 1 1 1
  spline S23 degree 3 poles (61.1095, 13.479) (60.1068, 13.8067) (60.4374, 15.1149) (61.1095, 15.1149) knots 0 0 0 0 1 1 1 1
  line L10 (61.1095, 15.1149) -> (61.1095, 13.479)
  line L11 (61.7956, 10.0849) -> (61.7956, 11.9291)
  spline S24 degree 3 poles (61.7956, 11.9291) (62.801, 11.7347) (62.7149, 10.2765) (61.7956, 10.0849) knots 0 0 0 0 1 1 1 1
  spline S25 degree 3 poles (148.6457, 10.5459) (148.5068, 10.7293) (148.4124, 10.9459) (148.3624, 11.1987) knots 0 0 0 0 1 1 1 1
  spline S26 degree 3 poles (149.7956, 9.0378) (150.4094, 9.1267) (150.8899, 9.3655) (151.2343, 9.7571) knots 0 0 0 0 1 1 1 1
  spline S27 degree 3 poles (151.7509, 11.1987) (151.7509, 11.7097) (151.6148, 12.1263) (151.3398, 12.4541) knots 0 0 0 0 1 1 1 1
  spline S28 degree 3 poles (147.7819, 9.6238) (148.1235, 9.2822) (148.5651, 9.0794) (149.1095, 9.0156) knots 0 0 0 0 1 1 1 1
  line L12 (149.1095, 15.1149) -> (149.1095, 13.479)
  line L13 (149.1095, 12.1291) -> (149.1095, 10.1488)
  spline S29 degree 3 poles (149.7956, 11.9291) (150.801, 11.7347) (150.7149, 10.2765) (149.7956, 10.0849) knots 0 0 0 0 1 1 1 1
  line L14 (150.3622, 14.3428) -> (151.5565, 14.4983)
  line L15 (149.7956, 8.1545) -> (149.7956, 9.0378)
  spline S30 degree 3 poles (149.7956, 15.0983) (150.1011, 14.9649) (150.2899, 14.715) (150.3622, 14.3428) knots 0 0 0 0 1 1 1 1
  spline S31 degree 3 poles (147.318, 14.2317) (147.318, 13.7206) (147.4625, 13.2873) (147.7513, 12.929) knots 0 0 0 0 1 1 1 1
  spline S32 degree 3 poles (147.8069, 15.5343) (147.4819, 15.1844) (147.318, 14.7483) (147.318, 14.2317) knots 0 0 0 0 1 1 1 1
  spline S33 degree 3 poles (155.1117, 12.3846) (155.1117, 9.2572) (152.5675, 6.713) (149.44, 6.713) knots 0 0 0 0 1 1 1 1
  spline S34 degree 3 poles (149.44, 19.1895) (145.6876, 19.1895) (142.6352, 16.137) (142.6352, 12.3846) knots 0 0 0 0 1 1 1 1
  line L16 (148.3624, 11.1987) -> (147.1292, 11.0653)
  line L17 (149.7956, 16.1426) -> (149.7956, 16.6092)
  spline S35 degree 3 poles (151.5565, 14.4983) (151.4759, 14.9705) (151.2843, 15.3482) (150.9899, 15.6288) knots 0 0 0 0 1 1 1 1
  line L18 (149.1095, 9.0156) -> (149.1095, 8.1545)
  spline S36 degree 3 poles (149.1095, 16.1426) (148.5679, 16.0898) (148.1346, 15.8871) (147.8069, 15.5343) knots 0 0 0 0 1 1 1 1
  spline S37 degree 3 poles (149.44, 5.5798) (153.1924, 5.5798) (156.2449, 8.6323) (156.2449, 12.3846) knots 0 0 0 0 1 1 1 1
  spline S38 degree 3 poles (151.2343, 9.7571) (151.5787, 10.1488) (151.7509, 10.6293) (151.7509, 11.1987) knots 0 0 0 0 1 1 1 1
  spline S39 degree 3 poles (149.1095, 10.1488) (148.9401, 10.2293) (148.7845, 10.3626) (148.6457, 10.5459) knots 0 0 0 0 1 1 1 1
  spline S40 degree 3 poles (151.3398, 12.4541) (151.0649, 12.7818) (150.551, 13.0457) (149.7956, 13.2512) knots 0 0 0 0 1 1 1 1
  line L19 (149.7956, 13.2512) -> (149.7956, 15.0983)
  line L20 (149.7956, 10.0849) -> (149.7956, 11.9291)
  line L21 (149.1095, 8.1545) -> (149.7956, 8.1545)
  spline S41 degree 3 poles (149.44, 18.0563) (152.5675, 18.0563) (155.1117, 15.5121) (155.1117, 12.3846) knots 0 0 0 0 1 1 1 1
  spline S42 degree 3 poles (149.1095, 13.479) (148.1068, 13.8067) (148.4374, 15.1149) (149.1095, 15.1149) knots 0 0 0 0 1 1 1 1
  spline S43 degree 3 poles (150.9899, 15.6288) (150.6927, 15.9121) (150.2955, 16.0815) (149.7956, 16.1426) knots 0 0 0 0 1 1 1 1
  spline S44 degree 3 poles (147.1292, 11.0653) (147.2236, 10.446) (147.4402, 9.9655) (147.7819, 9.6238) knots 0 0 0 0 1 1 1 1
  line L22 (149.1095, 16.6092) -> (149.1095, 16.1426)
  spline S45 degree 3 poles (149.44, 6.713) (146.3126, 6.713) (143.7684, 9.2572) (143.7684, 12.3846) knots 0 0 0 0 1 1 1 1
  spline S46 degree 3 poles (142.6352, 12.3846) (142.6352, 8.6323) (145.6876, 5.5798) (149.44, 5.5798) knots 0 0 0 0 1 1 1 1
  spline S47 degree 3 poles (147.7513, 12.929) (148.0402, 12.5707) (148.4929, 12.3041) (149.1095, 12.1291) knots 0 0 0 0 1 1 1 1
  line L23 (149.7956, 16.6092) -> (149.1095, 16.6092)
  spline S48 degree 3 poles (156.2449, 12.3846) (156.2449, 16.137) (153.1924, 19.1895) (149.44, 19.1895) knots 0 0 0 0 1 1 1 1
  spline S49 degree 3 poles (143.7684, 12.3846) (143.7684, 15.5121) (146.3126, 18.0563) (149.44, 18.0563) knots 0 0 0 0 1 1 1 1
extrude "Extrude1" add sketch "Sketch3" along normal blind 0.4
extrude "Extrude2" add sketch "Sketch1" sketch "Sketch4" along normal blind 0.4 from surface at 0.4 of sketch 2
fillet "Fillet1" radius 7.5 4 edges at (166.5514, -1.6336, 0.2) (166.5514, 53.7573, 0.2) (46.9601, 53.7573, 0.2) (46.9601, -1.6336, 0.2)
